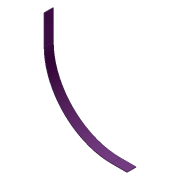
# Autodesk Inventor part: Shooter Curve
Saved by Autodesk Inventor 2012 (Build 160160000, 160)
## iProperties
Created: 2013-01-16
Part Number: Shooter Curve
Material: Default
Document SubType Name: Modeling
Designer: William
Density: 1 g/cm^3
Mass: 260.182 g
Surface Area: 928.357 cm^2
Volume: 260.182 cm^3
Author: William
Autodesk Inventor part; units mm, degrees
ref_plane "YZ Plane" through (0, 0, 0) normal (1, 0, 0) x (0, 1, 0)
ref_plane "XZ Plane" through (0, 0, 0) normal (0, 1, 0) x (-1, 0, 0)
ref_plane "XY Plane" through (0, 0, 0) normal (0, 0, 1) x (1, 0, 0)
sketch "Sketch1" plane through (0, 0, 0) normal (0, 0, 1) x (1, 0, 0)
  arc A0 (-5.2229, -27.1112) -> (369.4271, -401.7612) centre (369.4271, -27.1112) ccw
  arc A1 (-8.3979, -27.1112) -> (369.4271, -404.9362) centre (369.4271, -27.1112) ccw
  line L0 (-5.2229, -27.1112) -> (-5.2229, 138.3204)
  line L1 (-5.2229, 138.3204) -> (-8.3979, 138.3204)
  line L2 (-8.3979, 138.3204) -> (-8.3979, -27.1112)
  line L3 (369.4271, -404.9362) -> (457.1448, -404.9362)
  line L4 (457.1448, -404.9362) -> (457.1448, -401.7612)
  line L5 (457.1448, -401.7612) -> (369.4271, -401.7612)
  line L6 (-5.2229, -27.1112) -> (-8.3979, -27.1112) construction
  point P0 (0, 0)
  dimension "d0" = 749.3
  dimension "d2" = 3.175
  constraints: 14 end point, 4 point on circle, 4 tangent, 3 horizontal, 2 centre point, 2 parallel, 1 coincident, 1 perpendicular, 1 other
  measures "d0" diameter of A0
  measures "d2" distance of L1.end L0.end
extrude "Extrusion1" add sketch "Sketch1" along normal blind 50.8
body "Solid1"
